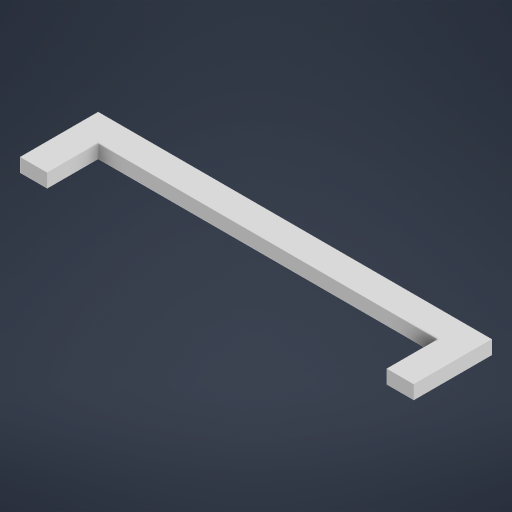
# Autodesk Inventor part: Langbektang houder
Saved by Autodesk Inventor 2023.2 (Build 272271000, 271)
## iProperties
Created: 2020-09-09
Part Number: Langbektang houder
Material: Generic
Document SubType Name: Modeling
Designer: nathan.bollaert
Density: 1 g/cm^3
Appearance: Default
Author: nathan.bollaert
Autodesk Inventor part; units mm, degrees
ref_plane "YZ Plane" through (0, 0, 0) normal (1, 0, 0) x (0, 1, 0)
ref_plane "XZ Plane" through (0, 0, 0) normal (0, 1, 0) x (-1, 0, 0)
ref_plane "XY Plane" through (0, 0, 0) normal (0, 0, 1) x (1, 0, 0)
sketch "Sketch1" plane through (0, 0, 0) normal (0, 1, 0) x (-1, 0, 0)
  line L0 (0, 0) -> (0, -15)
  line L1 (0, -15) -> (0, -23)
  line L2 (0, -23) -> (-116, -23)
  line L3 (-116, -23) -> (-116, -15)
  line L4 (-116, -15) -> (-116, 0)
  line L5 (-116, 0) -> (-108, 0)
  line L6 (-108, 0) -> (-108, -15)
  line L7 (-108, -15) -> (-8, -15)
  line L8 (-8, -15) -> (-8, 0)
  line L9 (-8, 0) -> (0, 0)
  dimension "d243" = 8
  dimension "d245" = 100
  dimension "d246" = 15
  constraints: 20 end point, 6 equal length, 5 perpendicular, 3 point on line, 1 vertical
  measures "d243" distance of L4.end L5.end
  measures "d245" distance of L6.end L7.end
  measures "d246" distance of L7.end L8.end
extrude "Extrusion1" add sketch "Sketch1" along normal blind 4
body "Solid5"
